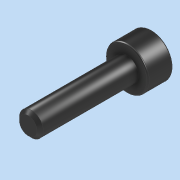
# Autodesk Inventor part: LUC GIAC
Saved by Autodesk Inventor 2021 (Build 250183000, 183)
## iProperties
Created: 2022-03-09
Part Number: LUC GIAC
Material: Generic
Document SubType Name: Modeling
Designer: 41601100
Density: 1 g/cm^3
Appearance: Default
Author: 41601100
Autodesk Inventor part; units mm, degrees
ref_plane "YZ Plane" through (0, 0, 0) normal (1, 0, 0) x (0, 1, 0)
ref_plane "XZ Plane" through (0, 0, 0) normal (0, 1, 0) x (-1, 0, 0)
ref_plane "XY Plane" through (0, 0, 0) normal (0, 0, 1) x (1, 0, 0)
sketch "Sketch1" plane through (0, 0, 0) normal (0, 0, 1) x (1, 0, 0)
  point P0 (0, 0)
sketch "Sketch2" plane through (0, 0, 0) normal (0, 0, 1) x (1, 0, 0)
  circle A0 centre (0, 0) radius 3.4
  dimension "d0" = 6.8
  constraints: 1 centre point, 1 coincident
  measures "d0" diameter of A0
extrude "Extrusion1" add sketch "Sketch2" along normal blind 4
sketch "Sketch3" plane through (0, 0, 4) normal (0, 0, 1) x (1, 0, 0)
  circle A0 centre (0, 0) radius 3.4 projected
  circle A1 centre (0, 0) radius 1.9
  dimension "d3" = 3.8
  constraints: 1 centre point, 1 coincident
  measures "d3" diameter of A1
extrude "Extrusion2" add sketch "Sketch3" along normal blind 15.7 contours A1
sketch "Sketch4" plane through (0, 0, 0) normal (0, 0, -1) x (-1, 0, 0)
  circle A0 centre (0, 0) radius 3.4 projected
  circle A1 centre (0, 0) radius 3.4 projected
  line L0 (-0.8625, 1.4939) -> (0.8625, 1.4939)
  line L1 (0.8625, 1.4939) -> (1.725, 0)
  line L2 (1.725, 0) -> (0.8625, -1.4939)
  line L3 (0.8625, -1.4939) -> (-0.8625, -1.4939)
  line L4 (-1.725, 0) -> (-0.8625, -1.4939)
  line L5 (-1.725, 0) -> (-0.8625, 1.4939)
  constraints: 12 end point, 2 parallel
extrude "Extrusion3" cut sketch "Sketch4" against normal blind 2.45 contours L0 L1 L2 L3 L4 L5
fillet "Fillet1" radius 0.2 6 edges at (1.2937, 0.7469, 0) (0, 1.4939, 0) (-1.2937, 0.7469, 0) (-1.2937, -0.7469, 0) (0, -1.4939, 0) (1.2937, -0.7469, 0)
fillet "Fillet2" radius 0.2 2 edges at (-3.4, 0, 0) (-3.4, 0, 4)
chamfer "Chamfer1" distance 0.5 angle 45 1 edges at (-1.9, 0, 19.7)
body "Solid1"
